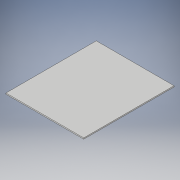
# Autodesk Inventor part: planche
Saved by Autodesk Inventor 2019 (Build 230136000, 136)
## iProperties
Created: 2018-11-20
Part Number: planche
Material: Générique
Document SubType Name: Modeling
Designer: pouey
Density: 1 g/cm^3
Appearance: Par défaut
Author: pouey
Autodesk Inventor part; units mm, degrees
ref_plane "YZ Plane" through (0, 0, 0) normal (1, 0, 0) x (0, 1, 0)
ref_plane "XZ Plane" through (0, 0, 0) normal (0, 1, 0) x (-1, 0, 0)
ref_plane "XY Plane" through (0, 0, 0) normal (0, 0, 1) x (1, 0, 0)
sketch "Esquisse1" plane through (0, 0, 0) normal (0, 1, 0) x (-1, 0, 0)
  line L0 (0, 0) -> (495, 0)
  line L1 (495, 0) -> (495, -495)
  line L2 (495, -495) -> (0, -495)
  line L3 (0, -495) -> (0, 0)
  dimension "d0" = 495
  dimension "d1" = 495
  constraints: 8 end point, 2 parallel, 1 horizontal, 1 perpendicular
  measures "d0" distance of L0.end L1.end
  measures "d1" distance of L1.end L2.end
extrude "Extrusion1" add sketch "Esquisse1" along normal blind 5
sketch "Esquisse2" plane through (0, 5, 0) normal (0, 1, 0) x (1, 0, 0)
  line L0 (0, 0) -> (0, 495) projected
  line L1 (0, 0) -> (-495, 0)
  line L2 (-495, 0) -> (-495, 100)
  line L3 (-495, 100) -> (0, 100)
  line L4 (0, 100) -> (0, 0)
  dimension "d4" = 495
  dimension "d5" = 100
  constraints: 8 end point, 2 parallel, 1 horizontal, 1 perpendicular
  measures "d4" distance of L2.end L3.end
  measures "d5" distance between parallel lines of L1 L3
extrude "Extrusion2" cut sketch "Esquisse2" against normal blind 5
sketch "Esquisse3" plane through (0, 5, 0) normal (0, 1, 0) x (1, 0, 0)
  line L0 (0, 100) -> (-495, 100) projected
  line L1 (0, 495) -> (-495, 495) projected
  line L2 (0, 100) -> (-155, 100)
  line L3 (-155, 100) -> (-155, 495)
  line L4 (-155, 495) -> (0, 495)
  line L5 (0, 495) -> (0, 100)
  point P0 (0, 0)
  dimension "d8" = 155
  constraints: 8 end point, 2 parallel, 1 horizontal, 1 perpendicular, 1 point on line
  measures "d8" distance between parallel lines of L5 L3
extrude "Extrusion3" cut sketch "Esquisse3" against normal blind 5
